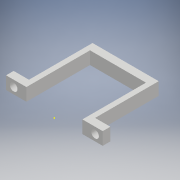
# Autodesk Inventor part: servo shaft
Saved by Autodesk Inventor 2017 (Build 210142000, 142)
## iProperties
Created: 2019-12-11
Part Number: servo shaft
Material: Generic
Document SubType Name: Modeling
Designer: User
Density: 1 g/cm^3
Appearance: Default
Author: User
Autodesk Inventor part; units mm, degrees
ref_plane "YZ Plane" through (0, 0, 0) normal (1, 0, 0) x (0, 1, 0)
ref_plane "XZ Plane" through (0, 0, 0) normal (0, 1, 0) x (-1, 0, 0)
ref_plane "XY Plane" through (0, 0, 0) normal (0, 0, 1) x (1, 0, 0)
sketch "Sketch1" plane through (0, 0, 0) normal (0, 0, 1) x (1, 0, 0)
  line L0 (-10, 25) -> (10, 25)
  line L1 (13, 28) -> (-13, 28)
  line L2 (-13, 28) -> (-13, 3)
  line L3 (13, 3) -> (13, 28)
  line L4 (11, 0) -> (17, 0)
  line L5 (17, 3) -> (13, 3)
  line L6 (-13, 3) -> (-17, 3)
  line L7 (-17, 0) -> (-11, 0)
  line L8 (-17, 3) -> (-19, 3)
  line L9 (-19, 3) -> (-19, 0)
  line L10 (-19, 0) -> (-17, 0)
  line L11 (17, 0) -> (19, 0)
  line L12 (19, 0) -> (19, 3)
  line L13 (17, 3) -> (19, 3)
  line L14 (-10, 25) -> (-11, 25)
  line L15 (-11, 25) -> (-11, 0)
  line L16 (10, 25) -> (11, 25)
  line L17 (11, 25) -> (11, 0)
  point P0 (0, 0)
  dimension "d0" = 20
  dimension "d2" = 3
  dimension "d12" = 3
  dimension "d17" = 1
  constraints: 36 end point, 7 perpendicular, 3 horizontal, 1 parallel, 1 point on line
  measures "d0" distance of L0.start L0.end
  measures "d2" distance between parallel lines of L0 L1
  measures "d12" distance of L11.end L12.end
  measures "d17" distance of L0.end L16.end
extrude "Extrusion1" add sketch "Sketch1" along normal blind 5
sketch "Sketch2" plane through (-19, 3, 0) normal (0, 1, 0) x (1, 0, 0)
  circle A0 centre (3, -2.5) radius 1.5
  point P0 (19, 0)
  dimension "d13" = 3
  constraints: 1 centre point
  measures "d13" diameter of A0
extrude "Extrusion2" cut sketch "Sketch2" against normal up to next
sketch "Sketch3" plane through (-13, 28, 0) normal (0, 1, 0) x (1, 0, 0)
  point P0 (13, 0)
mirror "Mirror1" about plane through (0, 0, 0) normal (1, 0, 0) of "Extrusion2"
sketch "Sketch4" plane through (-19, 0, 0) normal (0, -1, 0) x (1, 0, 0)
  point P0 (19, 0)
body "Solid1"
